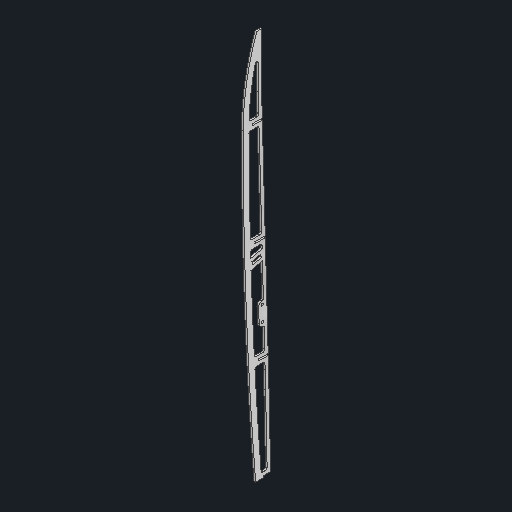
# Autodesk Inventor part: stringer_cowl
Saved by Autodesk Inventor 2023 (Build 270158030, 158C)
## iProperties
Created: 2022-03-23
Part Number: stringer_cowl
Material: Generic
Document SubType Name: Modeling
Designer: kardo
Density: 1 g/cm^3
Appearance: Default
Author: kardo
Autodesk Inventor part; units mm, degrees
ref_plane "YZ Plane" through (0, 0, 0) normal (1, 0, 0) x (0, 1, 0)
ref_plane "XZ Plane" through (0, 0, 0) normal (0, 1, 0) x (-1, 0, 0)
ref_plane "XY Plane" through (0, 0, 0) normal (0, 0, 1) x (1, 0, 0)
derived "parameters_frame.ipt"
derived "surface_body.ipt"
sketch "sk_rail_top_cowl" plane through (54.6, 0, 0) normal (1, 0, 0) x (0, 1, 0)
  spline S0 degree 2 poles (-363, 39.712) (-181.6483, 54.394) (0, 54.4) knots 0 0 0 1 1 1
  spline S1 degree 3 poles (0, 54.4) (31.284, 54.4) (68.256, 47.9917) (94.8, 37.536) knots 1 1 1 1 2 2 2 2
  point P0 (0, 0)
sketch "sk_rail_bottom_standoff" plane through (34.32, 0, 0) normal (1, 0, 0) x (0, 1, 0)
  line L0 (-363, 18.496) -> (-275.8801, 20.463)
  arc A0 (-275.8801, 20.463) -> (-254.1001, 21.0191) centre (-359.1231, 3707.4463) ccw
  line L1 (30.81, 28.832) -> (94.8, 28.832)
  arc A1 (30.81, 28.832) -> (9.48, 28.5282) centre (30.81, -720.1791) ccw
  line L2 (-254.1001, 21.0191) -> (9.48, 28.5282)
  line L3 (-483, 0) -> (357, 0) construction
  line L4 (9.48, 28.5282) -> (9.48, 0) construction
  line L5 (-254.1001, 21.0191) -> (-254.1001, 0) construction
  point P0 (0, 0)
  point P1 (-254.1001, 20.9547)
  point P2 (9.48, 28.832)
ref_plane "plane_middle" through (0, 0, 0) normal (0, 1, 0) x (-1, 0, 0)
ref_plane "plane_rear" through (0, -363, 0) normal (0, 1, 0) x (-1, 0, 0)
ref_plane "plane_cowl_right" through (54.6, 0, 0) normal (1, 0, 0) x (0, 1, 0)
ref_plane "plane_nose" through (0, 94.8, 0) normal (0, 1, 0) x (-1, 0, 0)
ref_plane "plane_tail_1" through (0, -120.9999, 0) normal (0, 1, 0) x (-1, 0, 0)
ref_plane "plane_tail_2" through (0, -242.0001, 0) normal (0, 1, 0) x (-1, 0, 0)
derived "stencil_frame.ipt"
sketch "sk_cowl_joint_locations" plane through (54.6, 0, 0) normal (1, 0, 0) x (0, 1, 0)
  line L0 (-363, 18.496) -> (-275.8801, 20.463) construction
  arc A0 (-275.8801, 20.463) -> (-254.1001, 21.0191) centre (-359.1231, 3707.4463) ccw construction
  line L1 (-254.1001, 21.0191) -> (9.48, 28.5282) construction
  arc A1 (30.81, 28.832) -> (9.48, 28.5282) centre (30.81, -720.1791) ccw construction
  line L2 (30.81, 28.832) -> (94.8, 28.832) construction
  line L3 (94.8, 30.032) -> (30.81, 30.032) construction
  arc A2 (30.81, 30.032) -> (9.4458, 29.7277) centre (30.81, -720.1791) ccw construction
  line L4 (9.4458, 29.7277) -> (-254.1343, 22.2186) construction
  arc A3 (-275.9072, 21.6626) -> (-254.1343, 22.2186) centre (-359.1231, 3707.4463) ccw construction
  line L5 (-275.9072, 21.6626) -> (-363, 19.6963) construction
  line L6 (-242.0001, 4666.1952) -> (-242.0001, -2045.0469) construction
  line L7 (-120.9999, 4666.1952) -> (-120.9999, -2045.0469) construction
  line L8 (-363, 4666.1952) -> (-363, -2045.0469) construction
  line L9 (0, 4666.1952) -> (0, -2045.0469) construction
  line L10 (-242.0001, 45.0688) -> (-242.0001, 22.5643) construction
  line L11 (-120.9999, 49.9661) -> (-120.9999, 26.0115) construction
  line L12 (-363, 19.6963) -> (-363, 19.6963)
  line L13 (-363, 19.6963) -> (-363, 36.9211) construction
  line L14 (-1246.9714, 4491.7596) -> (383.4376, -2047.4538) construction
  line L15 (-362.7741, 36.9211) -> (-363, 39.712) construction
  spline S0 degree 2 poles (-363, 39.712) (-181.6483, 54.394) (0, 54.4) knots 0 0 0 1 1 1
  spline S1 degree 3 poles (0, 54.4) (31.284, 54.4) (68.256, 47.9917) (94.8, 37.536) knots 1 1 1 1 2 2 2 2
  line L16 (0, 51.6) -> (0, 29.4586) construction
  spline S2 degree 3 poles (93.7738, 34.9308) (89.4268, 36.6431) (81.2968, 39.4556) (71.234, 42.2519) (63.4432, 44.1558) (58.1419, 45.3261) (51.4169, 46.6598) (45.9725, 47.6212) (39.1225, 48.6857) (33.6211, 49.4253) (26.7536, 50.2046) (21.2812, 50.7098) (14.5037, 51.1886) (7.8073, 51.5121) (2.5751, 51.6) (0, 51.6) knots 1 1 1 1 1.166667 1.291667 1.333333 1.416667 1.458333 1.541667 1.583333 1.666667 1.708333 1.791667 1.833333 1.916667 2 2 2 2
  spline S3 degree 3 poles (0, 51.6) (-20.1706, 51.5993) (-55.4643, 51.3605) (-95.7903, 50.6123) (-126.0307, 49.8474) (-146.1889, 49.2356) (-171.3841, 48.3435) (-191.5382, 47.528) (-216.7283, 46.3813) (-236.8783, 45.3621) (-262.0632, 43.9608) (-282.2091, 42.7379) (-307.3889, 41.082) (-332.5661, 39.2987) (-352.7052, 37.7363) (-362.7741, 36.9211) knots 0 0 0 0 0.166667 0.291667 0.333333 0.416667 0.458333 0.541667 0.583333 0.666666 0.708333 0.791666 0.833333 0.916666 1 1 1 1
  line L17 (-142.5135, 45.4866) -> (-137.5404, 25.5402) construction
  line L18 (-134.9025, 31.4945) -> (-138.7836, 30.5268) construction
  line L19 (-137.3891, 41.4677) -> (-141.2702, 40.5) construction
  line L20 (-142.5135, 45.4866) -> (-138.6324, 46.4543) construction
  line L21 (-137.5404, 25.5402) -> (-133.6592, 26.5079) construction
  line L22 (-138.6324, 46.4543) -> (-138.8117, 52.2515) construction
  point P0 (0, 0)
  point P1 (-363, 28.3087)
  point P2 (-242.0001, 33.8165)
  point P3 (-120.9999, 37.9888)
  point P4 (0, 40.5293)
  point P5 (-1246.9714, 4491.7596)
  point P6 (383.4376, -2047.4538)
  point P7 (-85.2629, 50.788)
  point P8 (0, 40.5293)
sketch "sk_servo_mount" plane through (-54.6, 0, 0) normal (1, 0, 0) x (0, 1, 0)
  line L0 (-254.1001, 21.0191) -> (9.48, 28.5282) construction
  line L1 (-363, 4666.1952) -> (-363, -2045.0469) construction
  line L2 (0, 4666.1952) -> (0, -2045.0469) construction
  line L3 (-204.8284, 22.4228) -> (-205.0163, 29.0201) construction
  line L4 (-205.0163, 29.0201) -> (-187.0237, 29.5327) construction
  line L5 (-187.0237, 29.5327) -> (-186.8357, 22.9354) construction
  point P0 (0, 0)
  point P1 (-196.02, 29.2764)
sketch "sk_base" plane through (54.6, 0, 0) normal (1, 0, 0) x (0, 1, 0)
  line L0 (-363, 18.496) -> (-275.8801, 20.463) construction
  arc A0 (-275.8801, 20.463) -> (-254.1001, 21.0191) centre (-359.1231, 3707.4463) ccw construction
  line L1 (-254.1001, 21.0191) -> (9.48, 28.5282) construction
  arc A1 (30.81, 28.832) -> (9.48, 28.5282) centre (30.81, -720.1791) ccw construction
  line L2 (30.81, 28.832) -> (94.8, 28.832) construction
  spline S0 degree 3 poles (0, 54.4) (31.284, 54.4) (68.256, 47.9917) (94.8, 37.536) knots 1 1 1 1 2 2 2 2 construction
  spline S1 degree 2 poles (-363, 39.712) (-181.6483, 54.394) (0, 54.4) knots 0 0 0 1 1 1 construction
  line L3 (-363, 4592.9714) -> (-363, -1605.7041) projected
  line L4 (94.8, 4592.9714) -> (94.8, -1605.7041) construction
  line L5 (92.8, 30.032) -> (30.81, 30.032)
  arc A2 (30.81, 30.032) -> (9.4458, 29.7277) centre (30.81, -720.1791) ccw
  line L6 (9.4458, 29.7277) -> (-254.1343, 22.2186)
  arc A3 (-275.9072, 21.6626) -> (-254.1343, 22.2186) centre (-359.1231, 3707.4463) ccw
  line L7 (-275.9072, 21.6626) -> (-363.0271, 19.6957)
  line L8 (92.8, 35.7395) -> (92.8, 30.032)
  line L9 (-363, 39.712) -> (-362.8063, 37.3198) construction
  line L10 (-362.8063, 37.3198) -> (-363, 37.3041)
  spline S2 degree 4 poles (-362.8063, 37.3198) (-272.302, 44.6469) (-181.601, 49.548) (-90.8004, 51.997) (0.0001, 52) knots 0 0 0 0 0 1 1 1 1 1
  spline S3 degree 5 poles (0, 52) (9.8053, 51.9997) (19.6091, 51.4715) (29.3793, 50.5419) (48.1612, 48.0094) (66.6851, 44.0076) (75.5322, 41.7141) (84.2786, 39.0221) (92.8, 35.7394) knots 0 0 0 0 0 0 0.517783 0.517783 0.517783 1 1 1 1 1 1
  point P0 (0, 0)
  point P1 (-363, 19.6963)
  dimension "d3" = 2.4
  dimension "d2" = 1.2
  dimension "d4" = 2
  constraints: 12 end point, 4 point on circle, 2 centre point, 1 parallel, 1 perpendicular, 1 point on line, 12 other
  measures "d2" distance between parallel lines of L1 L6
  measures "d4" distance between parallel lines of L4 L8
extrude "thicken" add sketch "sk_base" along normal blind 2
sketch "sk_cut_weight" plane through (54.6, 0, 0) normal (1, 0, 0) x (0, 1, 0)
  spline S0 degree 3 poles (-362.8063, 37.3198) (-352.7366, 38.1351) (-332.5957, 39.6976) (-307.4163, 41.481) (-282.2342, 43.1371) (-262.0865, 44.3602) (-236.8993, 45.7616) (-216.7476, 46.7809) (-191.5552, 47.9277) (-171.3993, 48.7432) (-146.2019, 49.6354) (-126.0419, 50.2472) (-95.7988, 51.0122) (-55.4692, 51.7605) (-20.1723, 51.9993) (0, 52) knots 0 0 0 0 0.083333 0.166667 0.208333 0.291667 0.333333 0.416667 0.458333 0.541667 0.583333 0.666667 0.708333 0.833333 1 1 1 1 construction
  line L0 (-275.9072, 21.6626) -> (-363.0271, 19.6957) construction
  line L1 (92.8, 35.7395) -> (92.8, 30.032) construction
  line L2 (-120.9999, 4592.9714) -> (-120.9999, -1605.7041) construction
  line L3 (-242.0001, 4592.9714) -> (-242.0001, -1605.7041) construction
  line L4 (-363, 4592.9714) -> (-363, -1605.7041) construction
  line L5 (0, 4592.9714) -> (0, -1605.7041) construction
  line L6 (9.4458, 29.7277) -> (-254.1343, 22.2186) construction
  arc A0 (-275.9072, 21.6626) -> (-254.1343, 22.2186) centre (-359.1231, 3707.4463) ccw construction
  line L7 (92.8, 30.032) -> (30.81, 30.032) construction
  arc A1 (30.81, 30.032) -> (9.4458, 29.7277) centre (30.81, -720.1791) ccw construction
  spline S1 degree 3 poles (0, 52) (2.5431, 52) (7.7084, 51.9144) (14.3167, 51.5995) (21.0044, 51.1333) (26.4043, 50.6413) (33.182, 49.8823) (38.6127, 49.1619) (45.3777, 48.1248) (50.7572, 47.1879) (57.4068, 45.8879) (62.653, 44.7468) (70.3708, 42.8898) (80.3553, 40.1612) (88.4545, 37.4138) (92.8, 35.7395) knots 1 1 1 1 1.08215 1.1643 1.205375 1.287525 1.3286 1.41075 1.451825 1.533975 1.57505 1.657199 1.698274 1.821499 1.985799 1.985799 1.985799 1.985799 construction
  line L8 (-361, 19.6957) -> (-361, 52) construction
  line L9 (-240.0001, 52) -> (-240.0001, 19.6957) construction
  line L10 (-118.9999, 52) -> (-118.9999, 19.6957) construction
  line L11 (2, 52) -> (2, 19.6957) construction
  line L12 (-357, 30.7639) -> (-357, 23.8328)
  line L13 (-246.0001, 26.4519) -> (-246.0001, 38.2412)
  line L14 (-236.0001, 38.7795) -> (-236.0001, 26.7368)
  line L15 (-114.9999, 43.5218) -> (-114.9999, 30.184)
  line L16 (-4, 33.3463) -> (-4, 44.9981)
  line L17 (6, 44.9206) -> (6, 33.6312)
  line L18 (75.9688, 34.032) -> (30.81, 34.032)
  arc A2 (30.81, 34.032) -> (9.3319, 33.7261) centre (30.81, -720.1791) ccw
  line L19 (9.3319, 33.7261) -> (-254.2482, 26.217)
  arc A3 (-275.9975, 25.6616) -> (-254.2482, 26.217) centre (-359.1231, 3707.4463) ccw
  line L20 (-275.9975, 25.6616) -> (-361, 23.7425)
  line L21 (-124.9999, 43.2538) -> (-124.9999, 29.8991)
  spline S2 degree 5 poles (75.9689, 34.032) (70.2355, 35.7235) (64.4443, 37.2192) (58.6145, 38.5504) (43.5097, 41.5782) (28.2329, 43.6133) (18.8435, 44.4966) (9.4225, 44.9996) (0, 45) knots 0 0 0 0 0 0 0.388161 0.388161 0.388161 1 1 1 1 1 1
  spline S3 degree 4 poles (0.0003, 45) (-90.3475, 44.997) (-180.6954, 42.5685) (-270.9449, 37.7087) (-361, 30.443) knots 0 0 0 0 0 1 1 1 1 1
  point P0 (0, 0)
  dimension "d51" = 7
  dimension "d18" = 2
  dimension "d19" = 2
  dimension "d20" = 2
  dimension "d21" = 2
  dimension "d22" = 4
  dimension "d23" = 4
  dimension "d26" = 4
  dimension "d27" = 4
  dimension "d28" = 4
  dimension "d29" = 4
  dimension "d30" = 4
  dimension "d52" = 4
  constraints: 28 end point, 11 parallel, 9 point on line, 8 horizontal alignment, 4 point on circle, 2 centre point, 17 other
  measures "d18" distance between parallel lines of L3 L9
  measures "d19" distance between parallel lines of L10 L2
  measures "d20" distance between parallel lines of L11 L5
  measures "d21" distance between parallel lines of L8 L4
  measures "d22" distance between parallel lines of L8 L12
  measures "d23" distance between parallel lines of L13 L3
  measures "d26" distance between parallel lines of L9 L14
  measures "d27" distance between parallel lines of L10 L15
  measures "d28" distance between parallel lines of L16 L5
  measures "d29" distance between parallel lines of L11 L17
  measures "d30" distance between parallel lines of L21 L2
  measures "d52" distance between parallel lines of L7 L18
extrude "cut_weight" cut sketch "sk_cut_weight" along normal through all both and the other way through all contours S3 L13 L19 A3 L20 L12 | S3 L21 L19 L14 | S3 L16 L19 L15 | L17 S2 L18 A2 L19
fillet "rounding" radius 2 15 edges at (55.6, -246.0001, 26.4519) (55.6, -124.9999, 29.8991) (55.6, -4, 33.3463) (55.6, 6, 33.6312) (55.6, -114.9999, 30.184) (55.6, -236.0001, 26.7368) (55.6, -357, 23.8328) (55.6, -357, 30.7639) (55.6, -236.0001, 38.7795) (55.6, -114.9999, 43.5218) (55.6, 6, 44.9206) (55.6, -4, 44.9981) (55.6, -124.9999, 43.2538) (55.6, -246.0001, 38.2412) (55.6, 75.9688, 34.032)
sketch "sk_joint_motor_mount" plane through (54.6, 0, 0) normal (1, 0, 0) x (0, 1, 0)
  spline S0 degree 3 poles (-362.8063, 37.3198) (-352.7366, 38.1351) (-332.5957, 39.6976) (-307.4163, 41.481) (-282.2342, 43.1371) (-262.0865, 44.3602) (-236.8993, 45.7616) (-216.7476, 46.7809) (-191.5552, 47.9277) (-171.3993, 48.7432) (-146.2019, 49.6354) (-126.0419, 50.2472) (-95.7988, 51.0122) (-55.4692, 51.7605) (-20.1723, 51.9993) (0, 52) knots 0 0 0 0 0.083333 0.166667 0.208333 0.291667 0.333333 0.416667 0.458333 0.541667 0.583333 0.666667 0.708333 0.833333 1 1 1 1 projected
  line L0 (9.4458, 29.7277) -> (-254.1343, 22.2186) projected
  line L1 (-137.3891, 41.4677) -> (-134.9025, 31.4945) construction
  line L2 (-137.3891, 41.4677) -> (-141.2702, 40.5) construction
  line L3 (-141.2702, 40.5) -> (-138.7836, 30.5268) construction
  line L4 (-138.7836, 30.5268) -> (-134.9025, 31.4945) construction
  line L5 (-147.6536, 49.568) -> (-141.6337, 25.4236)
  line L6 (-135.3828, 49.9552) -> (-129.3536, 25.7735)
  point P0 (0, 0)
  dimension "d33" = 4
  dimension "d34" = 4
  dimension "d35" = 4
  constraints: 12 end point, 3 parallel, 2 coincident, 2 perpendicular, 2 point on line, 2 other
  measures "d33" distance between parallel lines of L1 L3
  measures "d34" distance between parallel lines of L3 L5
  measures "d35" distance between parallel lines of L1 L6
extrude "joint_motor_mount" add sketch "sk_joint_motor_mount" along normal blind 2
sketch "sk_joint_servo" plane through (54.6, 0, 0) normal (1, 0, 0) x (0, 1, 0)
  line L0 (9.4458, 29.7277) -> (-254.1343, 22.2186) projected
  line L1 (-181.655, 24.2834) -> (-182.9099, 30.3795)
  arc A0 (-182.9099, 30.3795) -> (-187.1433, 33.731) centre (-187.0237, 29.5327) ccw
  line L2 (-187.1433, 33.731) -> (-205.136, 33.2184)
  arc A1 (-205.136, 33.2184) -> (-209.1716, 29.6313) centre (-205.0163, 29.0201) ccw
  line L3 (-209.1716, 29.6313) -> (-210.0774, 23.4737)
  point P0 (0, 0)
  dimension "d39" = 80
  dimension "d40" = 80
  dimension "d41" = 4.2
  constraints: 6 end point, 4 point on circle, 4 tangent, 2 centre point, 2 coincident, 2 point on line, 1 equal radius
  measures "d39" angle of L1 L0
  measures "d40" angle of L0 L3
  measures "d41" radius of A0
extrude "joint_servo" add sketch "sk_joint_servo" along normal blind 2
hole "drill_joint_servo" at (54.6, -205.0163, 29.0201) at (54.6, -187.0237, 29.5327) direction (1, 0, 0) diameter 3 end through all
sketch "sk_cowl_joint_cuts" plane through (54.6, 0, 0) normal (1, 0, 0) x (0, 1, 0)
  line L0 (-242.0001, 4592.9714) -> (-242.0001, -1605.7041) projected
  line L1 (-120.9999, 4592.9714) -> (-120.9999, -1605.7041) projected
  line L2 (0, 4592.9714) -> (0, -1605.7041) projected
  line L3 (-363, 4592.9714) -> (-363, -1605.7041) projected
  line L4 (-120.9999, -12.0112) -> (-118.9999, -12.0112)
  line L5 (-118.9999, -12.0112) -> (-118.9999, 37.9888)
  line L6 (-118.9999, 37.9888) -> (-120.9999, 37.9888)
  line L7 (0, -9.4707) -> (2, -9.4707)
  line L8 (2, -9.4707) -> (2, 40.5293)
  line L9 (2, 40.5293) -> (0, 40.5293)
  line L10 (-242.0001, 33.8165) -> (-240.0001, 33.8165)
  line L11 (-240.0001, 33.8165) -> (-240.0001, -16.1835)
  line L12 (-240.0001, -16.1835) -> (-242.0001, -16.1835)
  line L13 (-363, 28.3087) -> (-361, 28.3087)
  line L14 (-361, 28.3087) -> (-361, -21.6913)
  line L15 (-361, -21.6913) -> (-363, -21.6913)
  line L16 (-134.9025, 31.4945) -> (-137.3891, 41.4677)
  line L17 (-137.3891, 41.4677) -> (-141.2702, 40.5)
  line L18 (-141.2702, 40.5) -> (-138.7836, 30.5268)
  line L19 (-138.7836, 30.5268) -> (-134.9025, 31.4945)
  point P0 (0, 0)
  dimension "d8" = 2
  dimension "d15" = 50
  dimension "d16" = 4
  constraints: 33 end point, 11 parallel, 10 perpendicular, 4 point on line
  measures "d8" distance of L8.end L9.end
  measures "d15" distance of L7.end L8.end
  measures "d16" distance of L16.end L17.end
extrude "cut_joints" cut sketch "sk_cowl_joint_cuts" along normal through all
equation "\"d2\" = shell_thickness"
equation "\"d5\" = bulkhead_thickness"
equation "\"d51\" = bulkhead_inset + cowl_sealing_thickness"
equation "\"d18\" = bulkhead_thickness"
equation "\"d19\" = bulkhead_thickness"
equation "\"d20\" = bulkhead_thickness"
equation "\"d21\" = bulkhead_thickness"
equation "\"d22\" = bulkhead_inset"
equation "\"d23\" = bulkhead_inset"
equation "\"d26\" = bulkhead_inset"
equation "\"d27\" = bulkhead_inset"
equation "\"d28\" = bulkhead_inset"
equation "\"d29\" = bulkhead_inset"
equation "\"d30\" = bulkhead_inset"
equation "\"d38\" = 0.5 * bulkhead_inset"
equation "\"d33\" = 2 * bulkhead_thickness"
equation "\"d34\" = bulkhead_inset"
equation "\"d35\" = bulkhead_inset"
equation "\"d36\" = bulkhead_thickness"
equation "\"d41\" = 1.4 * drill_servo_mount_diam"
equation "\"d42\" = bulkhead_thickness"
equation "\"d44\" = drill_servo_mount_diam"
equation "\"d8\" = bulkhead_thickness"
equation "\"d16\" = 2 * bulkhead_thickness"
equation "\"shell_thickness\" = 1.2"
equation "\"bulkhead_thickness\" = 2"
equation "\"bulkhead_inset\" = 4"
equation "\"cowl_sealing_thickness\" = 3"
equation "\"drill_servo_mount_diam\" = 3"
body "Solid1"
